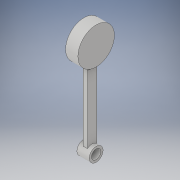
# Autodesk Inventor part: pendulum
Saved by Autodesk Inventor 2017.1 (Build 211199000, 199)
## iProperties
Created: 2017-05-25
Part Number: pendulum
Material: Generic
Document SubType Name: Modeling
Designer: 196918
Density: 1 g/cm^3
Appearance: Default
Author: 196918
Autodesk Inventor part; units mm, degrees
ref_plane "YZ Plane" through (0, 0, 0) normal (1, 0, 0) x (0, 1, 0)
ref_plane "XZ Plane" through (0, 0, 0) normal (0, 1, 0) x (-1, 0, 0)
ref_plane "XY Plane" through (0, 0, 0) normal (0, 0, 1) x (1, 0, 0)
sketch "Sketch1" plane through (0, 0, 0) normal (1, 0, 0) x (0, 1, 0)
  line L0 (9.8672, 30.93) -> (-65.8248, 30.93)
  line L1 (-65.8248, 30.93) -> (-65.8248, 21.786)
  line L2 (-65.8248, 21.786) -> (9.8672, 21.786)
  line L3 (9.8672, 21.786) -> (9.8672, 30.93)
  circle A0 centre (-65.8248, 26.358) radius 4.572
  circle A1 centre (-65.8248, 26.358) radius 6.8324
  point P0 (0, 0)
  dimension "d0" = 75.692
  dimension "d1" = 9.144
  constraints: 8 end point, 2 parallel, 1 centre point, 1 coincident, 1 horizontal, 1 midpoint, 1 perpendicular, 1 vertical alignment, 2 other
  measures "d0" distance of L2.end L1.end
  measures "d1" distance of L1.end L0.end
extrude "Extrusion3" add sketch "Sketch1" along normal mid plane 4.064 contours L3 L2 A1 L0 | A1 L2 A0 L0 | A0 L1 picked at (-59.8517, 25.4679) picked at (-64.4517, 25.6968)
extrude "Extrusion4" add sketch "Sketch1" along normal mid plane 12.192 contours A1 L2 A0 L0 | L0 A0 L2 A1
extrude "Extrusion5" cut sketch "Sketch1" along normal mid plane 12.192 contours A0 L1 | L1 A0
ref_plane "Work Plane1" through (0, 0, 0) normal (1, 0, 0) x (0, 0, -1)
sketch "Sketch2" plane through (0, 0, 0) normal (1, 0, 0) x (0, 0, -1)
  line L0 (-30.93, 9.8672) -> (-21.786, 9.8672) projected
  line L1 (-26.358, 9.8672) -> (-26.358, 27.0122)
  circle A0 centre (-26.358, 27.0122) radius 18.034
  point P0 (0, 0)
  dimension "d12" = 17.145
  dimension "d13" = 36.068
  constraints: 2 end point, 1 centre point, 1 coincident, 1 midpoint, 1 vertical
  measures "d12" distance of L1.start L1.end
  measures "d13" diameter of A0
extrude "Extrusion6" add sketch "Sketch2" along normal mid plane 12.192
fillet "Fillet1" radius 3.175 2 edges at (2.032, 8.9782, 26.358) (-2.032, 8.9782, 26.358)
body "Solid2"
